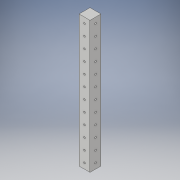
# Autodesk Inventor part: Frame 10
Saved by Autodesk Inventor 2018 (Build 220112000, 112)
## iProperties
Created: 2018-02-03
Part Number: Frame 10
Material: Generic
Document SubType Name: Modeling
Designer: kalra.rohan
Density: 1 g/cm^3
Appearance: Default
Author: kalra.rohan
Autodesk Inventor part; units mm, degrees
ref_plane "YZ Plane" through (0, 0, 0) normal (1, 0, 0) x (0, 1, 0)
ref_plane "XZ Plane" through (0, 0, 0) normal (0, 1, 0) x (-1, 0, 0)
ref_plane "XY Plane" through (0, 0, 0) normal (0, 0, 1) x (1, 0, 0)
sketch "Sketch1" plane through (0, 0, 0) normal (0, 0, 1) x (1, 0, 0)
  line L0 (0, 0) -> (25.4, 0)
  line L1 (25.4, 0) -> (25.4, -304.8)
  line L2 (25.4, -304.8) -> (0, -304.8)
  line L3 (0, -304.8) -> (0, 0)
  dimension "d0" = 304.8
  dimension "d1" = 25.4
  constraints: 8 end point, 2 parallel, 1 horizontal, 1 perpendicular
  measures "d0" distance between parallel lines of L2 L0
  measures "d1" distance between parallel lines of L1 L3
extrude "Extrusion1" add sketch "Sketch1" against normal blind 25.4
sketch "Sketch2" plane through (0, 0, 0) normal (0, 0, 1) x (1, 0, 0)
  circle A0 centre (12.7, -12.7) radius 1.9685
  line L0 (25.4, 0) -> (25.4, -304.8) projected
  line L1 (0, 0) -> (25.4, 0) projected
  circle A1 centre (12.7, -38.1) radius 1.9685
  circle A2 centre (12.7, -63.5) radius 1.9685
  circle A3 centre (12.7, -88.9) radius 1.9685
  circle A4 centre (12.7, -114.3) radius 1.9685
  circle A5 centre (12.7, -139.7) radius 1.9685
  circle A6 centre (12.7, -165.1) radius 1.9685
  circle A7 centre (12.7, -190.5) radius 1.9685
  circle A8 centre (12.7, -215.9) radius 1.9685
  circle A9 centre (12.7, -241.3) radius 1.9685
  circle A10 centre (12.7, -266.7) radius 1.9685
  circle A11 centre (12.7, -292.1) radius 1.9685
  dimension "d5" = 3.937
  dimension "d6" = 12.7
  dimension "d7" = 12.7
  dimension "d10" = 25.4
  constraints: 12 centre point, 1 vertical, 22 other
  measures "d5" diameter of A0
  measures "d6" distance from line of L0 A0.centre
  measures "d7" distance from line of A0.centre L1
  measures "d10" distance of A0.centre A1.centre
extrude "Extrusion2" cut sketch "Sketch2" against normal blind 304.8
sketch "Sketch3" plane through (25.4, -304.8, 0) normal (1, 0, 0) x (0, 0, -1)
  circle A0 centre (12.7, 292.1) radius 1.9685
  line L0 (0, 304.8) -> (25.4, 304.8) projected
  line L1 (25.4, 304.8) -> (25.4, 0) projected
  circle A1 centre (12.7, 266.7) radius 1.9685
  circle A2 centre (12.7, 241.3) radius 1.9685
  circle A3 centre (12.7, 215.9) radius 1.9685
  circle A4 centre (12.7, 190.5) radius 1.9685
  circle A5 centre (12.7, 165.1) radius 1.9685
  circle A6 centre (12.7, 139.7) radius 1.9685
  circle A7 centre (12.7, 114.3) radius 1.9685
  circle A8 centre (12.7, 88.9) radius 1.9685
  circle A9 centre (12.7, 63.5) radius 1.9685
  circle A10 centre (12.7, 38.1) radius 1.9685
  circle A11 centre (12.7, 12.7) radius 1.9685
  dimension "d17" = 3.937
  dimension "d18" = 12.7
  dimension "d19" = 12.7
  dimension "d22" = 25.4
  constraints: 12 centre point, 1 vertical, 22 other
  measures "d17" diameter of A0
  measures "d18" distance from line of A0.centre L0
  measures "d19" distance from line of A0.centre L1
  measures "d22" distance of A0.centre A1.centre
extrude "Extrusion3" cut sketch "Sketch3" against normal blind 304.8
body "Solid1"
